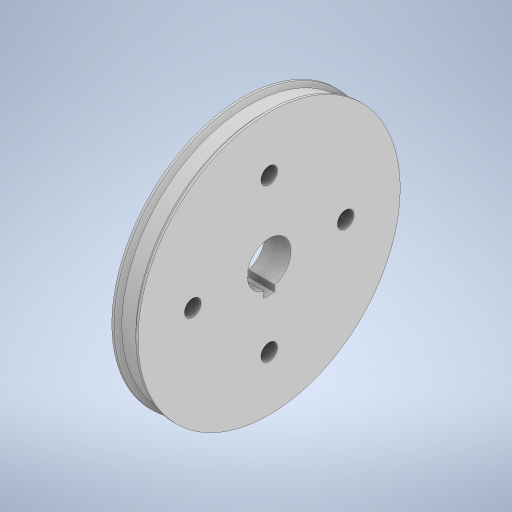
# Autodesk Inventor part: POLEA Pieza
Saved by Autodesk Inventor 2024 (Build 280153000, 153)
## iProperties
Created: 2024-02-06
Part Number: POLEA Pieza
Material: Genérico
Document SubType Name: Modeling
Designer: Andres
Density: 1 g/cm^3
Appearance: Valor por defecto
Author: Andres
Autodesk Inventor part; units mm, degrees
ref_plane "YZ Plane" through (0, 0, 0) normal (1, 0, 0) x (0, 1, 0)
ref_plane "XZ Plane" through (0, 0, 0) normal (0, 1, 0) x (-1, 0, 0)
ref_plane "XY Plane" through (0, 0, 0) normal (0, 0, 1) x (1, 0, 0)
sketch "Boceto1" plane through (0, 0, 0) normal (0, 0, 1) x (1, 0, 0)
  line L0 (0, 0) -> (0, 500)
  line L1 (100, 500) -> (100, 0)
  line L2 (100, 0) -> (0, 0)
  line L3 (0, 500) -> (17.6777, 482.3223)
  line L4 (100, 500) -> (82.3223, 482.3223)
  line L5 (82.3223, 482.3223) -> (17.6777, 482.3223)
  line L6 (50, -100) -> (-150, -100)
  constraints: 14 end point, 1 parallel, 1 perpendicular, 1 vertical
revolve "Revolución1" add sketch "Boceto1" angle 360 about axis through (50, -100, 0) along (-1, 0, 0)
sketch "Boceto2" plane through (100, -100, 0) normal (1, 0, 0) x (0, 0, -1)
  circle A0 centre (0, 0) radius 100 projected
  circle A1 centre (-350, 0) radius 37.5
  circle A2 centre (0, 350) radius 37.5
  circle A3 centre (350, 0) radius 37.5
  circle A4 centre (0, -350) radius 37.5
  point P0 (0, 100)
  dimension "d26" = 360
  constraints: 4 centre point, 1 vertical alignment, 9 other
extrude "Extrusión1" cut sketch "Boceto2" against normal blind 100 contours A1 | A2 | A3 | A4
thicken "Engrosado1" operation add thickness 10 both sides no extend neighbours no toward (1, 0, 0) faces at (100, -364.9419, 262.9039)
thicken "Engrosado2" operation add thickness 10 both sides no extend neighbours no toward (-1, 0, 0) faces at (0, -364.9419, 262.9039)
sketch "Boceto3" plane through (110, -100, 0) normal (1, 0, 0) x (0, 0, -1)
  line L0 (-25, -96.8246) -> (-25, -125)
  line L1 (-25, -125) -> (25, -125)
  line L2 (25, -125) -> (25, -96.8246)
  circle A0 centre (0, 0) radius 100 projected
  arc A1 (-25, -96.8246) -> (25, -96.8246) centre (0, 0) ccw
  point P0 (0, 100)
  point P1 (0, -100)
  constraints: 6 end point, 6 point on circle, 1 centre point, 1 coincident, 1 parallel
emboss "Repujado1" sketch "Boceto3" operation cut depth 120 direction (-1, 0, 0) contours A0 L2 L1 L0
